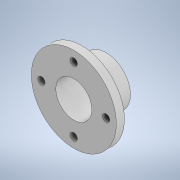
# Autodesk Inventor part: Cameralager21.8
Saved by Autodesk Inventor 2021 (Build 250183000, 183)
## iProperties
Created: 2022-06-27
Part Number: Cameralager21.8
Material: Generisch
Document SubType Name: Modeling
Designer: adria
Mass: 13.3722 g
Surface Area: 73.3957 cm^2
Volume: 13.3722 cm^3
Density: 1 g/cm^3
Appearance: Vorgabe
Author: adria
Autodesk Inventor part; units mm, degrees
ref_plane "YZ Plane" through (0, 0, 0) normal (1, 0, 0) x (0, 1, 0)
ref_plane "XZ Plane" through (0, 0, 0) normal (0, 1, 0) x (-1, 0, 0)
ref_plane "XY Plane" through (0, 0, 0) normal (0, 0, 1) x (1, 0, 0)
sketch "Skizze1" plane through (0, 0, 0) normal (0, 0, 1) x (1, 0, 0)
  circle A0 centre (0, 0) radius 15
  circle A1 centre (0, 0) radius 11.1
  dimension "d0" = 30
  dimension "d1" = 22.2
  constraints: 2 centre point, 1 coincident
  measures "d0" diameter of A0
  measures "d1" diameter of A1
extrude "Extrusion1" add sketch "Skizze1" along normal blind 20
sketch "Skizze2" plane through (0, 0, 20) normal (0, 0, 1) x (1, 0, 0)
  circle A0 centre (0, 0) radius 15 projected
  circle A1 centre (0, 0) radius 11.1 projected
  circle A2 centre (0, 0) radius 26.2393
  circle A3 centre (0, 0) radius 15
  constraints: 2 centre point, 2 coincident, 1 concentric
extrude "Extrusion2" add sketch "Skizze2" against normal blind 5 contours A2
sketch "Skizze3" plane through (0, 0, 20) normal (0, 0, 1) x (1, 0, 0)
  circle A0 centre (0, 0) radius 26.2393 projected
  line L0 (-36.7351, 0) -> (36.7351, 0) projected
  line L1 (0, -36.7351) -> (0, 36.7351) projected
  point P0 (0, 20)
  point P1 (-20, 0)
  point P2 (0, -20)
  point P3 (20, 0)
  dimension "d6" = 20
  dimension "d7" = 20
  dimension "d8" = 20
  dimension "d9" = 20
  constraints: 4 point on line
  measures "d6" distance of A0.centre point (0, 20)
  measures "d7" distance of A0.centre point (20, 0)
  measures "d8" distance of A0.centre point (0, -20)
  measures "d9" distance of A0.centre point (-20, 0)
hole "Bohrung1" at (0, 20, 20) at (-20, 0, 20) at (0, -20, 20) at (20, 0, 20) direction (0, 0, -1) diameter 4.4 end through all
